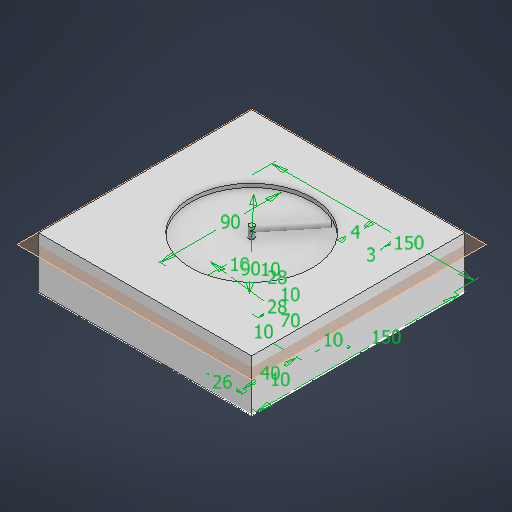
# Autodesk Inventor part: GPS-Compass-casing
Saved by Autodesk Inventor 2026.1 (Build 301233000, 233)
## iProperties
Created: 2025-07-21
Part Number: GPS-Compass-casing
Material: Generic
Document SubType Name: Modeling
Designer: MenMe
Density: 1 g/cm^3
Appearance: Default
Author: MenMe
Autodesk Inventor part; units mm, degrees
ref_plane "YZ Plane" through (0, 0, 0) normal (1, 0, 0) x (0, 1, 0)
ref_plane "XZ Plane" through (0, 0, 0) normal (0, 1, 0) x (-1, 0, 0)
ref_plane "XY Plane" through (0, 0, 0) normal (0, 0, 1) x (1, 0, 0)
sketch "Sketch1" plane through (0, 0, 0) normal (0, 1, 0) x (-1, 0, 0)
  line L0 (-75, 75) -> (75, 75)
  line L1 (75, 75) -> (75, -75)
  line L2 (75, -75) -> (-75, -75)
  line L3 (-75, -75) -> (-75, 75)
  line L4 (-75, 75) -> (75, -75) construction
  line L5 (75, 75) -> (-75, -75) construction
  line L6 (14, 14) -> (-14, 14)
  line L7 (-14, 14) -> (-14, -14)
  line L8 (-14, -14) -> (14, -14)
  line L9 (14, -14) -> (14, 14)
  line L10 (14, 14) -> (-14, -14) construction
  line L11 (-14, 14) -> (14, -14) construction
  circle A0 centre (0, 0) radius 35
  line L12 (-79, -79) -> (79, -79)
  line L13 (79, -79) -> (79, 79)
  line L14 (79, 79) -> (-79, 79)
  line L15 (-79, 79) -> (-79, -79)
  dimension "d0" = 150
  dimension "d1" = 150
  dimension "d2" = 28
  dimension "d3" = 28
  dimension "d4" = 70
  dimension "d7" = 4
  constraints: 32 end point, 6 parallel, 4 midpoint, 3 perpendicular, 2 horizontal, 1 centre point, 1 coincident, 3 other
  measures "d0" distance of L2.end L0.start
  measures "d1" distance of L1.end L2.end
  measures "d2" distance of L8.end L7.end
  measures "d3" distance of L7.end L6.end
  measures "d4" diameter of A0
  measures "d7" distance between parallel lines of L2 L12
extrude "Extrusion2" add sketch "Sketch1" along normal blind 35 contours L15 L14 L13 L12
extrude "Extrusion3" add sketch "Sketch1" along normal blind 3 contours L0 L1 L2 L3 | L9 L8 L7 L6 | A0
sketch "Sketch2" plane through (0, 3, 0) normal (0, 1, 0) x (1, 0, 0)
  line L0 (-14, -14) -> (14, -14)
  line L1 (14, -14) -> (14, 14)
  line L2 (14, 14) -> (-14, 14)
  line L3 (-14, 14) -> (-14, -14)
  line L4 (-14, -14) -> (14, 14) construction
  line L5 (14, -14) -> (-14, 14) construction
  point P0 (0, 0)
  dimension "d12" = 28
  dimension "d13" = 28
  constraints: 12 end point, 2 midpoint, 2 parallel, 1 horizontal, 1 perpendicular
  measures "d12" distance of L2.end L1.end
  measures "d13" distance of L1.end L0.end
extrude "Extrusion4" add sketch "Sketch2" along normal blind 28
sketch "Sketch3" plane through (0, 31, 0) normal (0, 1, 0) x (1, 0, 0)
  circle A0 centre (0, 0) radius 2
  dimension "d16" = 4
  constraints: 1 centre point, 1 coincident
  measures "d16" diameter of A0
extrude "Extrusion5" add sketch "Sketch3" along normal blind 12
sketch "Sketch4" plane through (0, 3, 0) normal (0, 1, 0) x (1, 0, 0)
  line L0 (-65, 72) -> (65, 72)
  line L1 (65, 72) -> (65, -18)
  line L2 (65, -18) -> (24, -18)
  line L3 (24, -18) -> (24, 24)
  line L4 (24, 24) -> (-24, 24)
  line L5 (-24, 24) -> (-24, -18)
  line L6 (-24, -18) -> (-65, -18)
  line L7 (-65, -18) -> (-65, 72)
  line L8 (-75, -75) -> (-75, 75) projected
  line L9 (75, 75) -> (75, -75) projected
  line L10 (-75, 75) -> (75, 75) projected
  line L11 (-14, 14) -> (14, 14) projected
  line L12 (-14, 14) -> (-14, -14) projected
  line L13 (14, 14) -> (14, -14) projected
  line L14 (39, -68) -> (65, -68)
  line L15 (65, -68) -> (65, -28)
  line L16 (65, -28) -> (39, -28)
  line L17 (39, -28) -> (39, -68)
  line L18 (-14, -14) -> (14, -14) projected
  point P0 (0, 0)
  point P1 (52, -28)
  point P2 (0, -14)
  dimension "d20" = 10
  dimension "d21" = 3
  dimension "d22" = 10
  dimension "d23" = 10
  dimension "d24" = 10
  dimension "d25" = 90
  dimension "d26" = 40
  dimension "d29" = 26
  dimension "d30" = 10
  dimension "d31" = 10
  constraints: 24 end point, 6 perpendicular, 2 midpoint, 2 parallel, 2 point on line, 1 horizontal, 1 vertical
  measures "d20" distance between parallel lines of L9 L1
  measures "d21" distance between parallel lines of L10 L0
  measures "d22" distance between parallel lines of L11 L4
  measures "d23" distance between parallel lines of L12 L5
  measures "d24" distance between parallel lines of L13 L3
  measures "d25" distance between parallel lines of L0 L6
  measures "d26" distance of L15.end L14.end
  measures "d29" distance of L14.start L14.end
  measures "d30" distance between parallel lines of L9 L15
  measures "d31" distance from line of L2 point (52, -28)
sketch "Sketch5" plane through (0, 31, 0) normal (0, 1, 0) x (1, 0, 0)
  circle A0 centre (0, 0) radius 45
  circle A1 centre (0, 0) radius 2.5714
  dimension "d32" = 90
  constraints: 2 centre point, 2 coincident
  measures "d32" diameter of A0
sketch "Sketch6" plane through (0, 35, 0) normal (0, 1, 0) x (1, 0, 0)
  line L0 (79, 79) -> (-79, 79) projected
  line L1 (-79, 79) -> (-79, -79) projected
  line L2 (79, 79) -> (-79, 79)
  line L3 (-79, 79) -> (-79, -79)
  line L4 (-79, -79) -> (79, -79)
  line L5 (79, -79) -> (79, 79)
  point P0 (0, 0)
  constraints: 8 end point, 2 parallel, 1 horizontal, 1 perpendicular
extrude "Extrusion6" add sketch "Sketch6" along normal blind 3
sketch "Sketch7" plane through (0, 38, 0) normal (0, 1, 0) x (1, 0, 0)
  circle A0 centre (0, 0) radius 2 projected
  circle A1 centre (0, 0) radius 45
  circle A2 centre (0, 0) radius 2.7692
  dimension "d42" = 90
  constraints: 2 centre point, 2 coincident
  measures "d42" diameter of A1
extrude "Extrusion8" cut sketch "Sketch7" against normal blind 2.75 contours A1 | A2
ref_plane "Work Plane1" through (-14, 3, -14) normal (0.6320613, 0, -0.7749184) x (0, 1, 0)
sketch "Sketch8" plane through (-14, 3, -14) normal (0.6320613, 0, -0.7749184) x (0, 1, 0)
  circle A0 centre (37.5996, 19.6977) radius 2
  line L0 (32.25, 17.6977) -> (40, 17.6977) projected
  point P0 (-3, 19.6977)
  constraints: 1 centre point, 1 tangent
extrude "Extrusion9" add sketch "Sketch8" along normal blind 40 and the other way blind 2.625
ref_plane "Work Plane2" through (0, 30.5, 0) normal (0, 1, 0) x (1, 0, 0)
sketch "Sketch9" plane through (0, 30.5, 0) normal (0, 1, 0) x (1, 0, 0)
  point P0 (0, 0)
body "Solid1"
